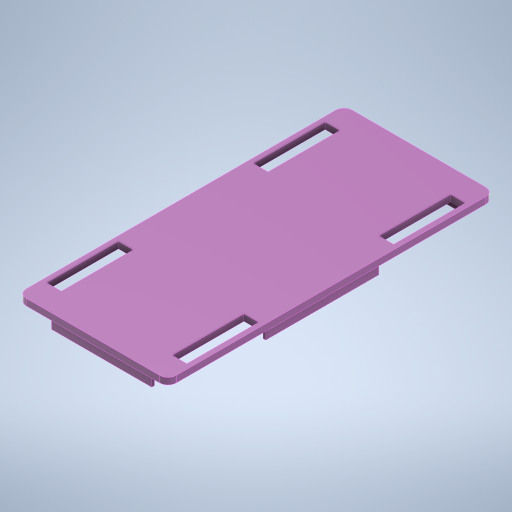
# Autodesk Inventor part: horni1
Saved by Autodesk Inventor 2023.2 (Build 272271000, 271)
## iProperties
Created: 2024-01-21
Part Number: horni1
Material: Generic
Document SubType Name: Modeling
Designer: marek
Density: 1 g/cm^3
Appearance: Smooth - Purple
Author: marek
Autodesk Inventor part; units mm, degrees
ref_plane "YZ Plane" through (0, 0, 0) normal (1, 0, 0) x (0, 1, 0)
ref_plane "XZ Plane" through (0, 0, 0) normal (0, 1, 0) x (-1, 0, 0)
ref_plane "XY Plane" through (0, 0, 0) normal (0, 0, 1) x (1, 0, 0)
sketch "Sketch1" plane through (0, 0, 0) normal (0, 1, 0) x (-1, 0, 0)
  line L0 (23, -50) -> (-23, -50)
  line L1 (-23, -50) -> (-23, 50)
  line L2 (-23, 50) -> (23, 50)
  line L3 (23, 50) -> (23, -50)
  line L4 (0, -70) -> (0, 70) projected
  line L5 (-32.2, 0) -> (32.2, 0) projected
  point P0 (0, 0)
  dimension "d0" = 46
  dimension "d1" = 100
  constraints: 8 end point, 2 parallel, 1 horizontal, 1 perpendicular, 2 other
  measures "d0" distance of L2.end L1.end
  measures "d1" distance of L1.end L0.end
extrude "Extrusion1" add sketch "Sketch1" along normal blind 2
fillet "Fillet1" radius 2.5 4 edges at (-23, 1, -50) (-23, 1, 50) (23, 1, -50) (23, 1, 50)
sketch "Sketch6" plane through (0, 0, 0) normal (0, -1, 0) x (1, 0, 0)
  line L0 (21.5, -42.7) -> (17, -42.7)
  line L1 (17, -42.7) -> (17, -20.7)
  line L2 (17, -20.7) -> (21.5, -20.7)
  line L3 (21.5, -20.7) -> (21.5, -42.7)
  line L4 (20.5, -50) -> (-20.5, -50) projected
  line L5 (23, 47.5) -> (23, -47.5) projected
  line L6 (0, 70) -> (0, -70) projected
  line L7 (-32.2, 0) -> (32.2, 0) projected
  line L8 (-21.5, -42.7) -> (-17, -42.7)
  line L9 (-17, -42.7) -> (-17, -20.7)
  line L10 (-17, -20.7) -> (-21.5, -20.7)
  line L11 (-21.5, -20.7) -> (-21.5, -42.7)
  line L12 (21.5, 42.7) -> (17, 42.7)
  line L13 (17, 42.7) -> (17, 20.7)
  line L14 (17, 20.7) -> (21.5, 20.7)
  line L15 (21.5, 20.7) -> (21.5, 42.7)
  line L16 (-21.5, 42.7) -> (-17, 42.7)
  line L17 (-17, 42.7) -> (-17, 20.7)
  line L18 (-17, 20.7) -> (-21.5, 20.7)
  line L19 (-21.5, 20.7) -> (-21.5, 42.7)
  point P0 (0, 0)
  dimension "d50" = 4.5
  dimension "d51" = 22
  dimension "d52" = 7.3
  dimension "d53" = 1.5
  constraints: 32 end point, 12 symmetric about line, 2 parallel, 1 horizontal, 1 perpendicular
  measures "d50" distance of L1.end L2.end
  measures "d51" distance of L0.end L1.end
  measures "d52" distance between parallel lines of L4 L0
  measures "d53" distance between parallel lines of L5 L3
extrude "Extrusion6" cut sketch "Sketch6" against normal through all
sketch "Sketch7" plane through (0, 0, 0) normal (0, -1, 0) x (1, 0, 0)
  line L0 (17, -20.7) -> (21.5, -20.7) projected
  line L1 (19.5, 17.35) -> (19.5, -17.35)
  line L2 (20.35, -17.35) -> (20.35, 17.35)
  line L3 (23, 47.5) -> (23, -47.5) projected
  line L4 (0, 70) -> (0, -70) projected
  line L5 (-32.2, 0) -> (32.2, 0) projected
  line L6 (21.5, 20.7) -> (17, 20.7) projected
  line L7 (15.35, 47.35) -> (-15.35, 47.35)
  line L8 (-15.35, 46.5) -> (15.35, 46.5)
  line L9 (-20.5, 50) -> (20.5, 50) projected
  line L10 (-15.371, 47.35) -> (-15.35, 47.35)
  line L11 (20.35, 17.35) -> (19.5, 17.35)
  line L12 (20.35, -17.35) -> (19.5, -17.35)
  line L13 (15.35, 46.5) -> (15.35, 47.35)
  line L14 (17, 20.7) -> (17, 42.7) projected
  line L15 (-15.35, 46.5) -> (-15.35, 47.35)
  line L16 (-17, 42.7) -> (-17, 20.7) projected
  line L17 (15.35, -47.35) -> (-15.35, -47.35)
  line L18 (-15.35, -46.5) -> (15.35, -46.5)
  line L19 (-15.371, -47.35) -> (-15.35, -47.35)
  line L20 (15.35, -46.5) -> (15.35, -47.35)
  line L21 (-15.35, -46.5) -> (-15.35, -47.35)
  line L22 (-17, -20.7) -> (-21.5, -20.7)
  line L23 (-19.5, 17.35) -> (-19.5, -17.35)
  line L24 (-20.35, -17.35) -> (-20.35, 17.35)
  line L25 (-21.5, 20.7) -> (-17, 20.7)
  line L26 (-20.35, 17.35) -> (-19.5, 17.35)
  line L27 (-20.35, -17.35) -> (-19.5, -17.35)
  line L28 (-23, -47.5) -> (-23, 47.5) projected
  point P0 (0, 0)
  dimension "d57" = 3.5
  dimension "d65" = 3.5
  dimension "d67" = 3.35
  dimension "d68" = 0.85
  dimension "d69" = 3.35
  dimension "d70" = 0.85
  dimension "d75" = 7.65
  dimension "d76" = 7.65
  constraints: 38 end point, 12 symmetric about line, 2 horizontal, 2 parallel, 2 perpendicular, 2 point on line, 2 vertical, 4 other
  measures "d57" distance between parallel lines of L3 L1
  measures "d65" distance between parallel lines of L9 L8
  measures "d68" distance between parallel lines of L1 L2
  measures "d69" distance between parallel lines of L0 L12
  measures "d70" distance between parallel lines of L7 L8
  measures "d75" distance between parallel lines of L13 L3
  measures "d76" distance between parallel lines of L28 L15
extrude "Extrusion7" add sketch "Sketch7" along normal blind 5
body "Solid1"
